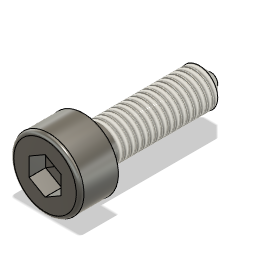
装配 (Autodesk Fusion 360 archive; units mm, degrees)
design "内六角头螺钉 ISO 4762 - M3 x 10 钢 4.6 平垫圈"
description: 内六角头螺钉 ISO 4762 - M3 x 10
Autodesk Fusion 360 part; units mm, degrees
sketch "Sketch1" plane through (0, 0, 0) normal (0, 1, 0) x (1, 0, 0)
  line L0 (-1.5, 0) -> (-1.5, 10)
  line L1 (-1.5, 10) -> (0, 10)
  line L2 (0, 10) -> (0, -3)
  line L3 (-1.5, 0) -> (-2.75, 0)
  line L4 (-2.75, 0) -> (-2.75, -3)
  line L5 (-2.75, -3) -> (0, -3)
  dimension "d9" = 3
  dimension "d66" = 5.5
  dimension "d68" = 10
  dimension "d79" = 3
  constraint perpendicular L0 L1
  constraint collinear origin L1.end L2.end
  constraint perpendicular L0 L3
  constraint coincident origin L3
  constraint vertical L0
  constraint vertical L2
  constraint parallel L2 L4
  constraint coincident L2 L5.end
  constraint perpendicular L2 L5
  measures "d68" distance of origin L1.end
  measures "d79" distance of L3.end L4.end
revolve "Revolve1" add sketch "Sketch1" angle 360 about axis through (0, 0, -10) along (0, 0, 1)
ref_plane "WorkPlane1" through (0, 0, 3) normal (0, 0, 1) x (1, 0, 0)
sketch "Sketch6" plane through (0, 0, 3) normal (0, 0, 1) x (1, 0, 0)
  line L0 (-1.25, 0) -> (1.25, 0) construction
  line L1 (0, 0) -> (-1.25, 0.7217)
  line L2 (-1.25, -0.7217) -> (-1.25, 0.7217)
  line L3 (-1.25, -0.7217) -> (0, 0)
  dimension "d72" = 2.5
  dimension "d104" = 150
  constraint horizontal L0
  constraint midpoint L1.start L0
  constraint coincident L1.start L3.end
  constraint perpendicular L0 L2
  constraint midpoint L0.start L2
  constraint coincident L1.end L2.end
  measures "d72" distance of L0.start L0.end
  measures "d104" angle of L0 L1
extrude "Extrude1" cut sketch "Sketch6" against normal blind 1.3
pattern_circular "C-Pattern1" count 6 over 360 about axis through (0, 0, 1.75) along (0, 0, 1) of "Extrude1"
extrude "Extrude2" cut 1 faces at (0, -0.4811, 1.7) along direction (0, 0, -1) blind 1.3 draft -85
fillet "Fillet4" radius 0.3 1 edges at (-2.5639, 0.9944, 3)
thread "Thread2" "ISO Metric profile 3.0 M3x0.5 6g" major diameter 2.927 minor diameter 2.3555 pitch 0.5 angle 60 resizes the face on face at (-1.4981, 0.0748, -3.3333) from (0, 0, -1.25) to (0, 0, -10)
sketch "Sketch7" plane through (0, 0, 0) normal (0, 1, 0) x (1, 0, 0)
  line L0 (-1.53, 10) -> (-1.53, 9)
  line L1 (-1.53, 9) -> (-0.53, 10)
  line L2 (0, 10) -> (0, -3)
  line L3 (-1.53, 10) -> (0, 10)
  dimension "d99" = 1.53
  dimension "d101" = 45
  dimension "d103" = 1
  constraint coincident L2.start L3.end
  constraint perpendicular L2 L3
  constraint coincident L1.end L3
  constraint perpendicular L0 L3
  measures "d99" distance of origin L0
  measures "d101" angle of L0 L1
  measures "d103" vertical distance of L0.end L1.end
revolve "Revolve3" cut sketch "Sketch7" angle 360 about axis through (0, 0, 1.75) along (0, 0, 1)
equation "d9 = adsk_nomdia"
equation "adsk_nomlen = 10.00 mm"
equation "adsk_headh = 3.00 mm"
equation "adsk_headdia = 5.50 mm"
equation "adsk_nomdia = 3.00 mm"
equation "adsk_waflat = 2.50 mm"
equation "d31 = -adsk_keyend"
equation "adsk_keyend = 1.30 mm"
equation "d66 = adsk_headdia"
equation "d68 = adsk_nomlen"
equation "d71 = adsk_headh"
equation "d72 = adsk_waflat"
equation "d76 = -adsk_keyend"
equation "d79 = adsk_headh"
equation "adsk_thrlen = 8.75 mm"
equation "d86 = adsk_nomdia * 0.1"
equation "d99 = adsk_nomdia * 0.51"
equation "adsk_fawi = 45.00 deg"
equation "d101 = adsk_fawi"
equation "adsk_pitch1 = 0.50 mm"
equation "d103 = 2 * adsk_pitch1"

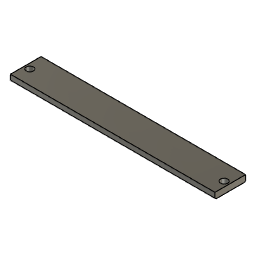
design "钢网夹盖"
Autodesk Fusion 360 part; units mm, degrees
sketch "草图1" plane through (0, 0, 0) normal (0, 0, 1) x (1, 0, 0)
  line L0 (0, 0) -> (100, 0)
  line L1 (100, 0) -> (100, 15)
  line L2 (100, 15) -> (0, 15)
  line L3 (0, 15) -> (0, 0)
  circle A0 centre (2.5, 7) radius 1.75
  circle A1 centre (97.5, 7) radius 1.75
  dimension "d1" = 100
  dimension "d2" = 15
  dimension "d3" = 3.5
  dimension "d4" = 3.5
  dimension "d5" = 7
  dimension "d6" = 7
  dimension "d7" = 2.5
  dimension "d8" = 2.5
  constraint horizontal L0
  constraint vertical L1
  constraint horizontal L2
  constraint vertical L3
  constraint coincident L0.start L3.end
  measures "d1" distance of L1.end L2.end
  measures "d2" distance of L0.start L2.end
  measures "d3" diameter of A0
  measures "d4" diameter of A1
  measures "d5" distance of L0 A0.centre
  measures "d6" distance of L0 A1.centre
  measures "d7" distance of L3 A0.centre
  measures "d8" distance of L1 A1.centre
extrude "拉伸1" add sketch "草图1" along normal blind 3
chamfer "倒角1" distance 0.5 angle 45 2 edges at (50, 0, 0) (50, 15, 0)

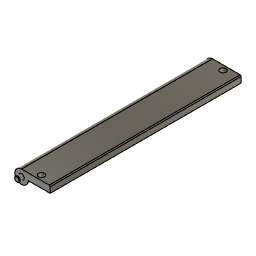
design "钢网夹座"
Autodesk Fusion 360 part; units mm, degrees
sketch "草图1" plane through (0, 0, 0) normal (0, 1, 0) x (1, 0, 0)
  circle A0 centre (0, 0) radius 3.5
  line L0 (0, 0) -> (15, 0)
  line L1 (15, 0) -> (15, -3.5)
  line L2 (15, -3.5) -> (0, -3.5)
  line L3 (0, -3.5) -> (0, 0)
  circle A1 centre (0, 0) radius 1.45
  dimension "d1" = 7
  dimension "d2" = 15
  dimension "d3" = 2.9
  constraint coincident A0.centre L0.start
  constraint horizontal L0
  constraint vertical L1
  constraint horizontal L2
  constraint vertical L3
  constraint tangent A0 L2
  measures "d1" diameter of A0
  measures "d2" distance of L1.end L2.end
  measures "d3" diameter of A1
extrude "拉伸1" add sketch "草图1" along normal blind 100
sketch "草图2" plane through (0, 0, 3.5) normal (0, 0, 1) x (-1, 0, 0)
  line L0 (0, 0) -> (-15, 0)
  line L1 (-15, 0) -> (-15, -100)
  line L2 (-15, -100) -> (0, -100)
  line L3 (0, -100) -> (0, 0)
  circle A0 centre (-8, -97.5) radius 1.6
  circle A1 centre (-8, -2.5) radius 1.6
  dimension "d6" = 3.2
  dimension "d7" = 7
  dimension "d8" = 2.5
  dimension "d9" = 3.2
  dimension "d10" = 7
  dimension "d11" = 2.5
  measures "d6" diameter of A0
  measures "d7" distance of L1 A0.centre
  measures "d8" distance of L2 A0.centre
  measures "d9" diameter of A1
  measures "d10" distance of L1 A1.centre
  measures "d11" distance of L0 A1.centre
extrude "拉伸2" cut sketch "草图2" against normal through all contours A0 | A1
extrude "拉伸3" add sketch "草图1" against normal blind 2.4 contours L0 L3 A1 | L0 L3 A1
sketch "草图3" plane through (0, 100, 0) normal (0, 1, 0) x (-1, 0, 0)
  arc A0 (-3.5, 0) -> (0, 3.5) centre (0, 0) ccw
  line L0 (0, 3.5) -> (-15, 3.5)
  line L1 (-15, 3.5) -> (-15, 0)
  line L2 (-15, 0) -> (-3.5, 0)
  circle A1 centre (0, 0) radius 1.45
  dimension "d15" = 2.9
  constraint coincident A0.centre A1.centre
  measures "d15" diameter of A1
extrude "拉伸4" add sketch "草图3" along normal blind 2.4 contours A1
chamfer "倒角1" distance 0.3 angle 45 2 edges at (1.3519, 102.4, -0.5243) (-1.3519, -2.4, -0.5243)
chamfer "倒角2" distance 0.5 angle 45 1 edges at (15, 50, 3.5)

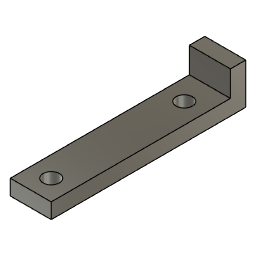
design "PCB限位"
Autodesk Fusion 360 part; units mm, degrees
sketch "草图1" plane through (0, 0, 0) normal (0, 0, 1) x (1, 0, 0)
  line L0 (0, 0) -> (8, 0)
  line L1 (8, 0) -> (8, 38)
  line L2 (8, 38) -> (0, 38)
  line L3 (0, 38) -> (0, 0)
  circle A0 centre (4, 4) radius 1.6
  circle A1 centre (4, 30) radius 1.6
  line L4 (4, 0) -> (4, 38) construction
  dimension "d1" = 38
  dimension "d2" = 8
  dimension "d3" = 3.2
  dimension "d4" = 3.2
  dimension "d5" = 4
  dimension "d6" = 8
  constraint horizontal L0
  constraint vertical L1
  constraint horizontal L2
  constraint vertical L3
  constraint coincident L0.start L3.end
  constraint midpoint L0 L4.start
  constraint midpoint L2 L4.end
  constraint coincident A1.centre L4
  constraint coincident A0.centre L4
  measures "d1" distance of L0.start L2.end
  measures "d2" distance of L0.start L0.end
  measures "d3" diameter of A0
  measures "d4" diameter of A1
  measures "d5" distance of L0 A0.centre
  measures "d6" distance of L2 A1.centre
extrude "拉伸1" add sketch "草图1" along normal blind 3
sketch "草图2" plane through (0, 0, 3) normal (0, 0, 1) x (-1, 0, 0)
  circle A0 centre (-4, -4) radius 1.6
  circle A1 centre (-4, -30) radius 1.6
  line L0 (0, -38) -> (0, 0)
  line L1 (0, 0) -> (-8, 0)
  line L2 (-8, 0) -> (-8, -38)
  line L3 (-8, -38) -> (0, -38)
  line L4 (0, -38) -> (-8, -38)
  line L5 (-8, -38) -> (-8, -35)
  line L6 (-8, -35) -> (0, -35)
  line L7 (0, -35) -> (0, -38)
  dimension "d9" = 3
  constraint horizontal L4
  constraint vertical L5
  constraint horizontal L6
  constraint vertical L7
  constraint coincident L0.start L3.end
  measures "d9" distance of L0.start L6.end
extrude "拉伸2" add sketch "草图2" along normal blind 5 contours L0 L2 L3 L4 L5 L6 L7

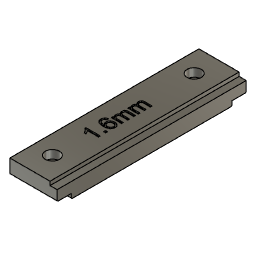
design "PCB夹具-板厚1.6mm"
Autodesk Fusion 360 part; units mm, degrees
sketch "草图1" plane through (0, 0, 0) normal (0, 0, 1) x (1, 0, 0)
  line L0 (0, 0) -> (20, 0)
  line L1 (20, 0) -> (20, 80)
  line L2 (20, 80) -> (0, 80)
  line L3 (0, 80) -> (0, 0)
  dimension "d1" = 20
  dimension "d2" = 80
  constraint horizontal L0
  constraint vertical L1
  constraint horizontal L2
  constraint vertical L3
  constraint coincident L0.start L3.end
  measures "d1" distance of L0.start L0.end
  measures "d2" distance of L0.start L2.end
extrude "拉伸1" add sketch "草图1" along normal blind 6.4
sketch "草图2" plane through (0, 0, 6.4) normal (0, 0, 1) x (-1, 0, 0)
  line L0 (0, -80) -> (0, 0)
  line L1 (0, 0) -> (-20, 0)
  line L2 (-20, 0) -> (-20, -80)
  line L3 (-20, -80) -> (0, -80)
  line L4 (0, -80) -> (-17, -80)
  line L5 (-17, -80) -> (-17, 0)
  line L6 (-17, 0) -> (0, 0)
  line L7 (0, 0) -> (0, -80)
  dimension "d8" = 17
  constraint horizontal L4
  constraint vertical L5
  constraint horizontal L6
  constraint vertical L7
  constraint coincident L1 L5.end
  constraint coincident L0.start L3.end
  measures "d8" distance of L0.start L4.end
extrude "拉伸2" add sketch "草图2" along normal blind 1.6 contours L0 L1 L3 L4 L5 L6 L7
sketch "草图3" plane through (0, 0, 8) normal (0, 0, 1) x (-1, 0, 0)
  line L0 (0, 0) -> (-17, 0)
  line L1 (-17, 0) -> (-17, -80)
  line L2 (-17, -80) -> (0, -80)
  line L3 (0, -80) -> (0, 0)
  line L4 (-8, -80) -> (-8, 0) construction
  circle A0 centre (-8, -70) radius 1.5
  circle A1 centre (-8, -10) radius 1.5
  dimension "d11" = 8
  dimension "d12" = 3
  dimension "d13" = 3
  dimension "d14" = 60
  dimension "d15" = 10
  constraint coincident L2 L4.start
  constraint coincident L0 L4.end
  constraint perpendicular L0 L4
  constraint coincident L4 A0.centre
  constraint coincident L4 A1.centre
  measures "d11" distance of L3 L4
  measures "d12" diameter of A0
  measures "d13" diameter of A1
  measures "d14" distance of A0.centre A1.centre
  measures "d15" distance of L4.start A0.centre
hole "孔1" at (8, 10, 8) direction (0, 0, -1) diameter 3.2 end through all counterbore diameter 6 counterbore depth 3.5
hole "孔2" at (8, 70, 8) direction (0, 0, -1) diameter 3.2 end through all counterbore diameter 6 counterbore depth 3.5
sketch "草图5" plane through (0, 0, 8) normal (0, 0, 1) x (-1, 0, 0)
  circle A0 centre (-8, -70) radius 3
  circle A1 centre (-8, -10) radius 3
  line L0 (0, 0) -> (-17, 0)
  line L1 (-17, 0) -> (-17, -80)
  line L2 (-17, -80) -> (0, -80)
  line L3 (0, -80) -> (0, 0)
  line L4 (-11, -25) -> (-11, -53) construction
  line L5 (-11, -53) -> (-5, -53) construction
  line L6 (-5, -53) -> (-5, -25) construction
  line L7 (-5, -25) -> (-11, -25) construction
  dimension "d27" = 6
  dimension "d28" = 25
  dimension "d29" = 5
  text T0 "1.6mm" font "Arial" height 6 align left top in box 28 x 6 at (-11, -25) x (0, -1) y (1, 0) spacing 1 kerned
  measures "d28" distance of L0 L7
  measures "d29" distance of L3 L6
extrude "拉伸4" cut sketch "草图5" against normal blind 0.5 text T0
sketch "草图6" plane through (0, 0, 0) normal (0, 0, -1) x (1, 0, 0)
  circle A0 centre (8, -10) radius 1.6
  line L0 (0, 0) -> (0, -80)
  line L1 (0, -80) -> (20, -80)
  line L2 (20, -80) -> (20, 0)
  line L3 (20, 0) -> (0, 0)
  line L4 (0, 0) -> (20, 0)
  line L5 (20, 0) -> (20, -6)
  line L6 (20, -6) -> (0, -6)
  line L7 (0, -6) -> (0, 0)
  line L8 (0, -80) -> (20, -80)
  line L9 (20, -80) -> (20, -74)
  line L10 (20, -74) -> (0, -74)
  line L11 (0, -74) -> (0, -80)
  dimension "d32" = 6
  dimension "d33" = 6
  constraint horizontal L4
  constraint vertical L5
  constraint horizontal L6
  constraint vertical L7
  constraint coincident L2 L5.end
  constraint coincident L0.start L3.end
  constraint horizontal L8
  constraint vertical L9
  constraint horizontal L10
  constraint vertical L11
  constraint coincident L2 L9.end
  constraint coincident L0.end L1.start
  measures "d32" distance of L0.start L6.end
  measures "d33" distance of L0.end L10.end
extrude "拉伸5" cut sketch "草图6" against normal blind 2 contours L0 L2 L3 L4 L5 L6 L7 | L0 L1 L2 L8 L9 L10 L11
chamfer "倒角1" distance 0.3 angle 45 4 edges at (10, 0, 2) (10, 6, 0) (10, 80, 2) (10, 74, 0)

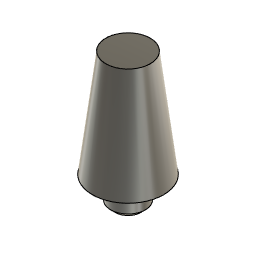
design "垫"
Autodesk Fusion 360 part; units mm, degrees
sketch "草图1" plane through (0, 0, 0) normal (0, 0, 1) x (1, 0, 0)
  circle A0 centre (0, 0) radius 4
  dimension "d1" = 8
  constraint coincident A0.centre origin
  measures "d1" diameter of A0
ref_plane "工作平面1" through (0, 0, 12) normal (0, 0, 1) x (1, 0, 0)
sketch "草图2" plane through (0, 0, 12) normal (0, 0, 1) x (1, 0, 0)
  circle A0 centre (0, 0) radius 2.5
  dimension "d3" = 5
  constraint coincident A0.centre origin
  measures "d3" diameter of A0
loft "放样1" add profiles "草图1", "草图2" section 1 section 2
sketch "草图4" plane through (0, 0, 0) normal (0, 0, -1) x (1, 0, 0)
  circle A0 centre (0, 0) radius 4
  circle A1 centre (0, 0) radius 1.95
  dimension "d4" = 3.9
  constraint concentric A0 A1
  measures "d4" diameter of A1
extrude "拉伸1" add sketch "草图4" along normal blind 3 contours A1
chamfer "倒角1" distance 0.5 angle 45 1 edges at (-1.818, 0.7052, -3)

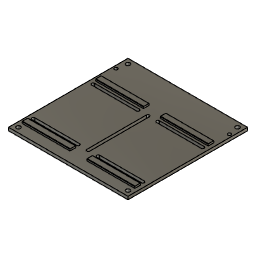
design "底板"
Autodesk Fusion 360 part; units mm, degrees
sketch "草图1" plane through (0, 0, 0) normal (0, 0, 1) x (1, 0, 0)
  line L0 (0, 0) -> (120, 0)
  line L1 (120, 0) -> (120, 120)
  line L2 (120, 120) -> (0, 120)
  line L3 (0, 120) -> (0, 0)
  line L4 (5, 78.5) -> (50, 78.5)
  arc A0 (50, 78.5) -> (50, 81.5) centre (50, 80) ccw
  line L5 (50, 81.5) -> (5, 81.5)
  arc A1 (5, 81.5) -> (5, 78.5) centre (5, 80) ccw
  line L6 (5, 80) -> (50, 80) construction
  line L7 (0, 50) -> (120, 50) construction
  line L8 (60, 120) -> (60, 0) construction
  line L9 (50, 18.5) -> (5, 18.5)
  arc A2 (5, 21.5) -> (5, 18.5) centre (5, 20) ccw
  line L10 (5, 21.5) -> (50, 21.5)
  arc A3 (50, 18.5) -> (50, 21.5) centre (50, 20) ccw
  line L11 (70, 81.5) -> (115, 81.5)
  arc A4 (115, 78.5) -> (115, 81.5) centre (115, 80) ccw
  line L12 (115, 78.5) -> (70, 78.5)
  arc A5 (70, 81.5) -> (70, 78.5) centre (70, 80) ccw
  line L13 (115, 21.5) -> (70, 21.5)
  arc A6 (115, 18.5) -> (115, 21.5) centre (115, 20) ccw
  line L14 (70, 18.5) -> (115, 18.5)
  arc A7 (70, 21.5) -> (70, 18.5) centre (70, 20) ccw
  circle A8 centre (5, 115) radius 2.05
  circle A9 centre (5, 5) radius 2.05
  circle A10 centre (115, 115) radius 2.05
  circle A11 centre (115, 5) radius 2.05
  line L15 (0, 104.95) -> (120, 104.95) construction
  circle A12 centre (3, 104.95) radius 1.6
  circle A13 centre (117, 104.95) radius 1.6
  line L16 (58.5, 80) -> (58.5, 20)
  arc A14 (58.5, 20) -> (61.5, 20) centre (60, 20) ccw
  line L17 (61.5, 20) -> (61.5, 80)
  arc A15 (61.5, 80) -> (58.5, 80) centre (60, 80) ccw
  line L18 (60, 80) -> (60, 20) construction
  point P0 (60, 120)
  dimension "d1" = 120
  dimension "d2" = 120
  dimension "d3" = 45
  dimension "d4" = 1.5
  dimension "d5" = 50
  dimension "d6" = 60
  dimension "d7" = 20
  dimension "d8" = 4.1
  dimension "d9" = 4.1
  dimension "d10" = 5
  dimension "d11" = 5
  dimension "d12" = 5
  dimension "d13" = 5
  dimension "d16" = 23.45
  dimension "d17" = 3.2
  dimension "d18" = 3
  dimension "d19" = 3.2
  dimension "d20" = 3
  dimension "d21" = 1.5
  dimension "d22" = 60
  dimension "d23" = 30
  constraint horizontal L0
  constraint vertical L1
  constraint horizontal L2
  constraint vertical L3
  constraint coincident L0.start L3.end
  constraint tangent L4 A0
  constraint tangent A0 L5
  constraint parallel L4 L5
  constraint tangent L5 A1
  constraint tangent L4 A1
  constraint horizontal L6
  constraint coincident L3 L7.start
  constraint coincident L1 L7.end
  constraint perpendicular L1 L7
  constraint coincident L2 P0
  constraint coincident L0 L8.end
  constraint perpendicular L0 L8
  constraint midpoint L2 P0
  constraint coincident L8 P0
  constraint symmetric L4.start L7 A2.start
  constraint symmetric L4.end L7 L10.end
  constraint symmetric A0.end L7 L9.start
  constraint symmetric L5.end L7 L9.end
  constraint symmetric A0 L7 A3
  constraint symmetric A1 L7 A2
  constraint symmetric L4.start L8 A4.start
  constraint symmetric L4.end L8 L12.end
  constraint symmetric A0.end L8 L11.start
  constraint symmetric L5.end L8 L11.end
  constraint symmetric A0 L8 A5
  constraint symmetric A1 L8 A4
  constraint symmetric L8 L9.start L14.start
  constraint symmetric L8 L9.end A6.start
  constraint symmetric L8 A2.start L13.start
  constraint symmetric L8 A2 A6
  constraint symmetric L8 L10.end L13.end
  constraint symmetric L8 A3 A7
  constraint symmetric L8 A8 A10
  constraint symmetric L8 A9 A11
  constraint coincident L3 L15.start
  constraint coincident L1 L15.end
  constraint perpendicular L1 L15
  constraint coincident L15 A12.centre
  constraint coincident L15 A13.centre
  constraint tangent L16 A14
  constraint tangent A14 L17
  constraint parallel L16 L17
  constraint tangent L17 A15
  constraint tangent L16 A15
  constraint coincident L8 A14.centre
  constraint parallel L8 L18
  measures "d1" distance of L0.start L0.end
  measures "d2" distance of L0.start L2.end
  measures "d3" distance of A1.centre A0.centre
  measures "d4" radius of A1
  measures "d5" distance of L0 L7
  measures "d6" distance of A1.centre A2.centre
  measures "d7" distance of A0.centre A5.centre
  measures "d8" diameter of A8
  measures "d9" diameter of A9
  measures "d10" distance of L2 A8.centre
  measures "d11" distance of L3 A8.centre
  measures "d12" distance of L3 A9.centre
  measures "d13" distance of L0 A9.centre
  measures "d16" distance of L5 L15
  measures "d17" diameter of A12
  measures "d18" distance of L3 A12.centre
  measures "d19" diameter of A13
  measures "d20" distance of L1 A13.centre
  measures "d21" radius of A15
  measures "d22" distance of A14.end L17.end
  measures "d23" distance of L7 A15.centre
extrude "拉伸1" add sketch "草图1" along normal blind 3
sketch "草图2" plane through (0, 0, 3) normal (0, 0, 1) x (-1, 0, 0)
  arc A0 (-5, -81.5) -> (-5, -78.5) centre (-5, -80) ccw
  line L0 (-5, -81.5) -> (-50, -81.5)
  arc A1 (-50, -78.5) -> (-50, -81.5) centre (-50, -80) ccw
  line L1 (-50, -78.5) -> (-5, -78.5)
  arc A2 (-61.5, -80) -> (-58.5, -80) centre (-60, -80) ccw
  line L2 (-61.5, -80) -> (-61.5, -20)
  arc A3 (-58.5, -20) -> (-61.5, -20) centre (-60, -20) ccw
  line L3 (-58.5, -20) -> (-58.5, -80)
  circle A4 centre (-117, -104.95) radius 1.6
  circle A5 centre (-3, -104.95) radius 1.6
  circle A6 centre (-115, -5) radius 2.05
  circle A7 centre (-5, -115) radius 2.05
  circle A8 centre (-5, -5) radius 2.05
  arc A9 (-70, -21.5) -> (-70, -18.5) centre (-70, -20) ccw
  line L4 (-70, -21.5) -> (-115, -21.5)
  arc A10 (-115, -18.5) -> (-115, -21.5) centre (-115, -20) ccw
  line L5 (-115, -18.5) -> (-70, -18.5)
  circle A11 centre (-115, -115) radius 2.05
  arc A12 (-115, -78.5) -> (-115, -81.5) centre (-115, -80) ccw
  line L6 (-115, -78.5) -> (-70, -78.5)
  arc A13 (-70, -81.5) -> (-70, -78.5) centre (-70, -80) ccw
  line L7 (-70, -81.5) -> (-115, -81.5)
  arc A14 (-5, -21.5) -> (-5, -18.5) centre (-5, -20) ccw
  line L8 (-5, -21.5) -> (-50, -21.5)
  arc A15 (-50, -18.5) -> (-50, -21.5) centre (-50, -20) ccw
  line L9 (-50, -18.5) -> (-5, -18.5)
  line L10 (0, -120) -> (0, 0)
  line L11 (0, 0) -> (-120, 0)
  line L12 (-120, 0) -> (-120, -120)
  line L13 (-120, -120) -> (0, -120)
  line L14 (-3.5, -89.75) -> (-51.5, -89.75)
  line L15 (-51.5, -89.75) -> (-51.5, -83.95)
  line L16 (-51.5, -83.95) -> (-3.5, -83.95)
  line L17 (-3.5, -83.95) -> (-3.5, -89.75)
  line L18 (-60, -120) -> (-60, 0) construction
  line L19 (-120, -50) -> (0, -50) construction
  line L20 (-116.5, -89.75) -> (-68.5, -89.75)
  line L21 (-116.5, -83.95) -> (-116.5, -89.75)
  line L22 (-68.5, -83.95) -> (-116.5, -83.95)
  line L23 (-68.5, -89.75) -> (-68.5, -83.95)
  line L24 (-3.5, -10.25) -> (-51.5, -10.25)
  line L25 (-3.5, -16.05) -> (-3.5, -10.25)
  line L26 (-51.5, -16.05) -> (-3.5, -16.05)
  line L27 (-51.5, -10.25) -> (-51.5, -16.05)
  line L28 (-68.5, -10.25) -> (-68.5, -16.05)
  line L29 (-116.5, -10.25) -> (-68.5, -10.25)
  line L30 (-68.5, -16.05) -> (-116.5, -16.05)
  line L31 (-116.5, -16.05) -> (-116.5, -10.25)
  point P0 (-61.5, -50)
  dimension "d24" = 2.45
  dimension "d25" = 5.8
  constraint horizontal L14
  constraint vertical L15
  constraint horizontal L16
  constraint vertical L17
  constraint tangent A0 L17
  constraint tangent A1 L15
  constraint midpoint L13 L18.start
  constraint midpoint L11 L18.end
  constraint coincident L12 L19.start
  constraint coincident L10 L19.end
  constraint perpendicular L10 L19
  constraint midpoint L2 P0
  constraint coincident L19 P0
  constraint symmetric L14.start L18 L20.start
  constraint symmetric L14.end L18 L20.end
  constraint symmetric L15.end L18 L22.start
  constraint symmetric L16.end L18 L21.start
  constraint symmetric L14.start L19 L24.start
  constraint symmetric L14.end L19 L24.end
  constraint symmetric L15.end L19 L26.start
  constraint symmetric L16.end L19 L25.start
  constraint symmetric L19 L20.start L29.start
  constraint symmetric L19 L20.end L28.start
  constraint symmetric L19 L21.start L30.end
  constraint symmetric L19 L22.start L28.end
  measures "d24" distance of L0 L16
  measures "d25" distance of L14.start L16.end
extrude "拉伸2" add sketch "草图2" along normal blind 1.8 contours L14 L15 L16 L17 | L20 L21 L22 L23 | L24 L25 L26 L27 | L28 L29 L30 L31
chamfer "倒角2" distance 0.3 angle 45 8 edges at (27.5, 83.95, 4.8) (27.5, 89.75, 4.8) (92.5, 89.75, 4.8) (92.5, 83.95, 4.8) (92.5, 16.05, 4.8) (92.5, 10.25, 4.8) (27.5, 16.05, 4.8) (27.5, 10.25, 4.8)
equation "d16 = 8.45 mm + 15 mm"

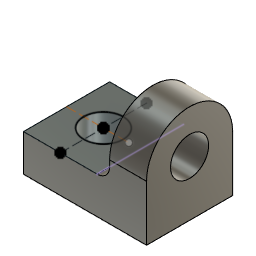
design "连杆固定座"
Autodesk Fusion 360 part; units mm, degrees
sketch "草图1" plane through (0, 0, 0) normal (1, 0, 0) x (0, 1, 0)
  line L0 (0, 0) -> (7, 0)
  line L1 (7, 0) -> (7, 4.5)
  line L2 (7, 4.5) -> (0, 4.5)
  line L3 (0, 4.5) -> (0, 0)
  circle A0 centre (3.5, 4.5) radius 3.5
  dimension "d4" = 4.5
  dimension "d5" = 7
  constraint horizontal L0
  constraint vertical L1
  constraint horizontal L2
  constraint vertical L3
  constraint coincident L0.start L3.end
  constraint midpoint L2 A0.centre
  constraint coincident L1.end A0
  measures "d4" distance of L0.end L1.end
  measures "d5" diameter of A0
extrude "拉伸1" add sketch "草图1" along normal blind 3
sketch "草图2" plane through (0, 0, 0) normal (0, -1, 0) x (1, 0, 0)
  line L0 (0, 0) -> (3, 0)
  line L1 (3, 0) -> (3, 4.5)
  line L2 (3, 4.5) -> (0, 4.5)
  line L3 (0, 0) -> (-7, 0)
  line L4 (-7, 0) -> (-7, 3)
  line L5 (-7, 3) -> (-1, 3)
  line L6 (0, 4) -> (0, 4.5)
  arc A0 (-1, 3) -> (0, 4) centre (-1, 4) ccw
  dimension "d11" = 3
  dimension "d13" = 7
  dimension "d20" = 1
  constraint horizontal L3
  constraint vertical L4
  constraint horizontal L5
  constraint coincident L0.start L3.start
  constraint coincident L2.end L6.end
  constraint perpendicular L2 L6
  constraint tangent L5 A0
  constraint tangent L6 A0
  measures "d11" distance of L3.end L4.end
  measures "d13" distance of L0.start L3.end
  measures "d20" radius of A0
extrude "拉伸2" add sketch "草图2" against normal up to surface (7 mm away)
sketch "草图3" plane through (0, 0, 3) normal (0, 0, 1) x (-1, 0, 0)
  line L0 (1, -7) -> (7, -7)
  line L1 (7, -7) -> (7, 0)
  line L2 (7, 0) -> (1, 0)
  line L3 (7, -3.5) -> (1.9365, -3.5) construction
  line L4 (4, -7) -> (4, 0) construction
  circle A0 centre (4, -3.5) radius 1.6
  line L5 (1, 0) -> (1, -7)
  point P0 (4, -3.5)
  dimension "d16" = 3
  dimension "d17" = 3.2
  constraint midpoint L1 L3.start
  constraint coincident L0 L4.start
  constraint coincident L2 L4.end
  constraint perpendicular L2 L4
  constraint midpoint L4 P0
  constraint coincident P0 A0.centre
  measures "d16" distance of L1 L4
  measures "d17" diameter of A0
extrude "拉伸4" cut sketch "草图3" against normal through all contours A0
sketch "草图4" plane through (3, 0, 0) normal (1, 0, 0) x (0, 1, 0)
  arc A0 (7, 4.5) -> (0, 4.5) centre (3.5, 4.5) ccw
  line L0 (0, 4.5) -> (0, 0)
  line L1 (0, 0) -> (7, 0)
  line L2 (7, 0) -> (7, 4.5)
  arc A1 (7, 4.5) -> (0, 4.5) centre (3.5, 4.5) ccw
  circle A2 centre (3.5, 4.5) radius 1.55
  dimension "d22" = 3.1
  constraint concentric A1 A2
  measures "d22" diameter of A2
extrude "拉伸5" cut sketch "草图4" against normal blind 2.5 contours A2

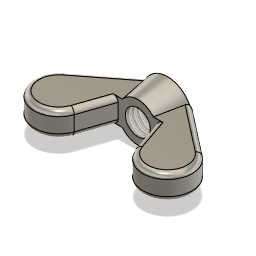
design "翼形螺母 JIS B 1185 - M3 钢 6 平垫圈"
description: 翼形螺母 JIS B 1185 - M3
Autodesk Fusion 360 part; units mm, degrees
sketch "Sketch1" plane through (0, 0, 0) normal (0, 1, 0) x (1, 0, 0)
  line L0 (0, 0) -> (0, -8)
  line L1 (0, -8) -> (8, -8) construction
  line L2 (8, -8) -> (8, 0) construction
  line L3 (0, 0) -> (2.5, 0)
  line L4 (0, -3) -> (2, -3)
  line L5 (2, -3) -> (2.5, 0)
  line L6 (1.5, 0) -> (1.5, -3)
  line L7 (5.5, -8) -> (5.5, -5.5) construction
  line L8 (8, -5.5) -> (5.5, -5.5) construction
  circle A0 centre (5.5, -5.5) radius 2.5
  line L9 (2.5, 0) -> (8, -4.277187)
  line L10 (2, -3) -> (3.714286, -8)
  point P0 (5.5, -8)
  point P1 (8, -5.5)
  dimension "d9" = 16
  dimension "d10" = 8
  dimension "d11" = 3
  dimension "d12" = 5
  dimension "d13" = 4
  dimension "d14" = 3
  dimension "d32" = 2.5
  dimension "d33" = 2.5
  dimension "d34" = 5
  constraint coincident L0.start L3.start
  constraint vertical L0
  constraint perpendicular L0 L1
  constraint parallel L0 L2
  constraint perpendicular L0 L3
  constraint perpendicular L0 L4
  constraint coincident L0 L4.start
  constraint coincident L2.end L3
  constraint parallel L0 L6
  constraint coincident L3 L6.start
  constraint coincident L4 L6.end
  constraint coincident L1 P0
  constraint coincident L2 P1
  constraint coincident P0 L7.start
  constraint perpendicular L1 L7
  constraint coincident P1 L8.start
  constraint perpendicular L2 L8
  constraint coincident L7.end L8.end
  constraint tangent A0 L10
  constraint tangent A0 L9
  measures "d10" distance of L1.end L2.end
  measures "d14" distance of L0.start L4.start
  measures "d32" distance of L1.end P0
  measures "d33" distance of L1.end P1
  measures "d34" diameter of A0
extrude "Extrude1" add sketch "Sketch1" along normal mid plane 2.5 contours L0 L3 L4 L6 | L3 L4 L5 L6 | L5 A0 L9 L10 | A0 picked at (1, -2) picked at (2, -1) picked at (2.950203, -2.093296) picked at (5.309366, -4.905033)
mirror "Mirror1" about plane through (0, 0, 0) normal (1, 0, 0) of bodies 1 merged
revolve "Revolve1" add sketch "Sketch1" angle 360 about axis through (0, 0, 0) along (0, 0, 1) contours L0 L3 L4 L6 | L3 L4 L5 L6 picked at (1, -2) picked at (2, -1)
revolve "Revolve2" cut sketch "Sketch1" angle 360 about axis through (0, 0, 0) along (0, 0, 1) contours L0 L3 L4 L6 picked at (1, -2)
thread "Thread1" "ISO Metric profile 3.0 M3x0.5 6H" major diameter 3.086 minor diameter 2.529 pitch 0.5 angle 60 resizes the face on face at (1.498135, -0.074769, 1)
chamfer "Chamfer1" distance 0.3 angle 30 1 edges at (-1.178928, -0.457263, 0) measured on face at (-2.088167, 0, 0)
fillet "Fillet2" radius 0.5 12 edges at (2.567569, 1.25, 4.655411) (6.952702, 1.25, 7.534614) (4.767369, 1.25, 1.763266) (-2.567569, 1.25, 4.655411) (-6.952702, 1.25, 7.534614) (-4.767369, 1.25, 1.763266) (-4.767369, -1.25, 1.763266) (-6.952702, -1.25, 7.534614) (-2.567569, -1.25, 4.655411) (4.767369, -1.25, 1.763266) (6.952702, -1.25, 7.534614) (2.567569, -1.25, 4.655411)
equation "adsk_nomdia = 3.00 mm"
equation "adsk_basedia = 5.00 mm"
equation "adsk_topdia = 4.00 mm"
equation "adsk_baseh = 3.00 mm"
equation "adsk_nheig = 8.00 mm"
equation "adsk_maxdia = 16.00 mm"
equation "adsk_wingrad = 2.50 mm"
equation "adsk_wingwidth = 2.50 mm"
equation "d9 = adsk_maxdia"
equation "d10 = adsk_nheig"
equation "d11 = adsk_nomdia"
equation "d12 = adsk_basedia"
equation "d13 = adsk_topdia"
equation "d14 = adsk_baseh"
equation "d16 = adsk_wingwidth"
equation "d24 = 0.1 * adsk_nomdia"
equation "d32 = adsk_wingrad"
equation "d33 = adsk_wingrad"
equation "d34 = adsk_wingrad * 2"
equation "d36 = 0.2 * adsk_wingwidth"

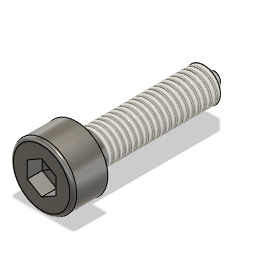
design "内六角头螺钉 ISO 4762 - M3 x 12 钢 4.6 平垫圈"
description: 内六角头螺钉 ISO 4762 - M3 x 12
Autodesk Fusion 360 part; units mm, degrees
sketch "Sketch1" plane through (0, 0, 0) normal (0, 1, 0) x (1, 0, 0)
  line L0 (-1.5, 0) -> (-1.5, 12)
  line L1 (-1.5, 12) -> (0, 12)
  line L2 (0, 12) -> (0, -3)
  line L3 (-1.5, 0) -> (-2.75, 0)
  line L4 (-2.75, 0) -> (-2.75, -3)
  line L5 (-2.75, -3) -> (0, -3)
  dimension "d9" = 3
  dimension "d66" = 5.5
  dimension "d68" = 12
  dimension "d79" = 3
  constraint perpendicular L0 L1
  constraint collinear origin L1.end L2.end
  constraint perpendicular L0 L3
  constraint coincident origin L3
  constraint vertical L0
  constraint vertical L2
  constraint parallel L2 L4
  constraint coincident L2 L5.end
  constraint perpendicular L2 L5
  measures "d68" distance of origin L1.end
  measures "d79" distance of L3.end L4.end
revolve "Revolve1" add sketch "Sketch1" angle 360 about axis through (0, 0, -12) along (0, 0, 1)
ref_plane "WorkPlane1" through (0, 0, 3) normal (0, 0, 1) x (1, 0, 0)
sketch "Sketch6" plane through (0, 0, 3) normal (0, 0, 1) x (1, 0, 0)
  line L0 (-1.25, 0) -> (1.25, 0) construction
  line L1 (0, 0) -> (-1.25, 0.7217)
  line L2 (-1.25, -0.7217) -> (-1.25, 0.7217)
  line L3 (-1.25, -0.7217) -> (0, 0)
  dimension "d72" = 2.5
  dimension "d104" = 150
  constraint horizontal L0
  constraint midpoint L1.start L0
  constraint coincident L1.start L3.end
  constraint perpendicular L0 L2
  constraint midpoint L0.start L2
  constraint coincident L1.end L2.end
  measures "d72" distance of L0.start L0.end
  measures "d104" angle of L0 L1
extrude "Extrude1" cut sketch "Sketch6" against normal blind 1.3
pattern_circular "C-Pattern1" count 6 over 360 about axis through (0, 0, 1.75) along (0, 0, 1) of "Extrude1"
extrude "Extrude2" cut 1 faces at (0, -0.4811, 1.7) along direction (0, 0, -1) blind 1.3 draft -85
fillet "Fillet4" radius 0.3 1 edges at (-2.5639, 0.9944, 3)
thread "Thread2" "ISO Metric profile 3.0 M3x0.5 6g" major diameter 2.927 minor diameter 2.3555 pitch 0.5 angle 60 resizes the face on face at (-1.4981, 0.0748, -4) from (0, 0, -1.25) to (0, 0, -12)
sketch "Sketch7" plane through (0, 0, 0) normal (0, 1, 0) x (1, 0, 0)
  line L0 (-1.53, 12) -> (-1.53, 11)
  line L1 (-1.53, 11) -> (-0.53, 12)
  line L2 (0, 12) -> (0, -3)
  line L3 (-1.53, 12) -> (0, 12)
  dimension "d99" = 1.53
  dimension "d101" = 45
  dimension "d103" = 1
  constraint coincident L2.start L3.end
  constraint perpendicular L2 L3
  constraint coincident L1.end L3
  constraint perpendicular L0 L3
  measures "d99" distance of origin L0
  measures "d101" angle of L0 L1
  measures "d103" vertical distance of L0.end L1.end
revolve "Revolve3" cut sketch "Sketch7" angle 360 about axis through (0, 0, 1.75) along (0, 0, 1)
equation "d9 = adsk_nomdia"
equation "adsk_nomlen = 12.00 mm"
equation "adsk_headh = 3.00 mm"
equation "adsk_headdia = 5.50 mm"
equation "adsk_nomdia = 3.00 mm"
equation "adsk_waflat = 2.50 mm"
equation "d31 = -adsk_keyend"
equation "adsk_keyend = 1.30 mm"
equation "d66 = adsk_headdia"
equation "d68 = adsk_nomlen"
equation "d71 = adsk_headh"
equation "d72 = adsk_waflat"
equation "d76 = -adsk_keyend"
equation "d79 = adsk_headh"
equation "adsk_thrlen = 10.75 mm"
equation "d86 = adsk_nomdia * 0.1"
equation "d99 = adsk_nomdia * 0.51"
equation "adsk_fawi = 45.00 deg"
equation "d101 = adsk_fawi"
equation "adsk_pitch1 = 0.50 mm"
equation "d103 = 2 * adsk_pitch1"
